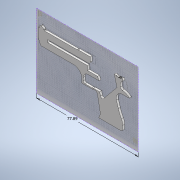
# Autodesk Inventor part: sheetmettaal_3
Saved by Autodesk Inventor 2022 (Build 260153000, 153)
## iProperties
Created: 2022-05-17
Part Number: sheetmettaal_3
Material: Generic
Document SubType Name: Sheet Metal
Designer: joshn
Density: 1 g/cm^3
Sheet Metal Rule: Default
Appearance: Default
Author: joshn
Autodesk Inventor part; units mm, degrees
ref_plane "YZ Plane" through (0, 0, 0) normal (1, 0, 0) x (0, 1, 0)
ref_plane "XZ Plane" through (0, 0, 0) normal (0, 1, 0) x (-1, 0, 0)
ref_plane "XY Plane" through (0, 0, 0) normal (0, 0, 1) x (1, 0, 0)
sketch "Sketch1" plane through (0, 0, 0) normal (0, 0, 1) x (1, 0, 0)
  line L0 (-5.5577, 9.6078) -> (72.3328, 9.6078) construction
  line L1 (72.3328, 9.6078) -> (72.3328, -46.9428) construction
  line L2 (72.3328, -46.9428) -> (-5.5577, -46.9428) construction
  line L3 (-5.5577, -46.9428) -> (-5.5577, 9.6078) construction
  point P0 (0, 0)
  dimension "d5" = 77.8905
  constraints: 1 vertical, 2 other
  measures "d5" distance of L1.end L2.end
sketch "Sketch2" plane through (0, 0, 0) normal (0, 0, 1) x (1, 0, 0)
  line L0 (1.7056, -0.1629) -> (1.7056, -0.6448)
  line L1 (-0.2664, 1.0493) -> (1.7056, -0.1629)
  line L2 (-0.7081, 1.0493) -> (-0.2664, 1.0493)
  arc A0 (-0.7081, 1.0493) -> (-1.4304, 0.327) centre (-0.7081, 0.327) ccw
  line L3 (-1.4304, -0.6448) -> (-1.4304, 0.327)
  line L4 (-2.6284, -0.6448) -> (-1.4304, -0.6448)
  line L5 (-2.6284, -7.7818) -> (-2.6284, -0.6448)
  line L6 (-0.8006, -12.1348) -> (-2.6284, -7.7818)
  line L7 (24.2675, -12.1348) -> (-0.8006, -12.1348)
  arc A1 (30.5055, -20.6992) -> (24.2675, -12.1348) centre (24.2675, -18.6888) ccw
  arc A2 (30.5055, -20.6992) -> (30.9333, -21.2865) centre (30.9333, -20.837) ccw
  line L8 (38.8712, -21.2865) -> (30.9333, -21.2865)
  line L9 (39.963, -20.923) -> (38.8712, -21.2865)
  arc A3 (42.6776, -22.7746) -> (39.963, -20.923) centre (40.3948, -23.2056) ccw
  line L10 (44.7723, -33.868) -> (42.6776, -22.7746)
  arc A4 (44.6306, -35.2789) -> (44.7723, -33.868) centre (42.2371, -34.3259) ccw
  line L11 (43.6296, -37.7931) -> (44.6306, -35.2789)
  line L12 (60.3255, -37.7931) -> (43.6296, -37.7931)
  line L13 (61.654, -37.1914) -> (60.3255, -37.7931)
  line L14 (61.8533, -33.7276) -> (61.654, -37.1914)
  arc A5 (61.8533, -33.7276) -> (60.9528, -29.7747) centre (54.5674, -33.3084) ccw
  arc A6 (58.6016, -24.1894) -> (60.9528, -29.7747) centre (85.7758, -16.0378) ccw
  line L15 (57.1367, -19.3061) -> (58.6016, -24.1894)
  arc A7 (61.717, -13.1502) -> (57.1367, -19.3061) centre (61.717, -17.9321) ccw
  line L16 (66.961, -13.1502) -> (61.717, -13.1502)
  arc A8 (66.961, -13.1502) -> (67.0884, -12.7993) centre (66.961, -12.9516) ccw
  arc A9 (67.0884, -12.7993) -> (61.7511, -10.5268) centre (60.666, -20.479) ccw
  arc A10 (60.1291, -9.1346) -> (61.7511, -10.5268) centre (61.9561, -8.647) ccw
  line L17 (59.0096, -4.9406) -> (60.1291, -9.1346)
  line L18 (55.449, -1.3577) -> (59.0096, -4.9406)
  line L19 (55.0519, -1.3577) -> (55.449, -1.3577)
  line L20 (57.6035, -10.735) -> (55.0519, -1.3577)
  line L21 (47.2749, -23.2615) -> (57.6035, -10.735)
  arc A11 (44.98, -22.7627) -> (47.2749, -23.2615) centre (46.2559, -22.4213) ccw
  line L22 (44.3049, -20.2402) -> (44.98, -22.7627)
  line L23 (33.0348, -20.5092) -> (36.1776, -20.5092)
  arc A12 (31.7579, -19.2323) -> (33.0348, -20.5092) centre (33.0348, -19.2323) ccw
  line L24 (31.7579, -17.0038) -> (31.7579, -19.2323)
  arc A13 (35.6115, -13.1502) -> (31.7579, -17.0038) centre (35.6115, -17.0038) ccw
  line L25 (36.1776, -13.1502) -> (35.6115, -13.1502)
  line L26 (42.6776, -10.735) -> (43.2318, -11.9426)
  line L27 (35.0069, -10.735) -> (42.6776, -10.735)
  line L28 (35.0069, -7.4885) -> (35.0069, -8.7654)
  line L29 (4.6149, -7.4885) -> (35.0069, -7.4885)
  line L30 (4.6149, -5.519) -> (4.6149, -7.4885)
  line L31 (35.7041, -5.519) -> (4.6149, -5.519)
  arc A14 (35.7041, -5.519) -> (37.089, -4.1341) centre (35.7041, -4.1341) ccw
  line L32 (37.089, -0.6448) -> (37.089, -4.1341)
  line L33 (28.0126, -0.6448) -> (37.089, -0.6448)
  arc A15 (27.0697, -0.9635) -> (28.0126, -0.6448) centre (27.0697, 0.5907) ccw
  line L34 (2.5258, -0.9635) -> (27.0697, -0.9635)
  arc A16 (1.9301, -0.6448) -> (2.5258, -0.9635) centre (2.5258, -0.2474) ccw
  line L35 (1.7056, -0.6448) -> (1.9301, -0.6448)
  arc A17 (38.0809, -13.3042) -> (39.1907, -13.9041) centre (40.5158, -10.1262) ccw
  arc A18 (38.0809, -13.3042) -> (37.6267, -13.1502) centre (37.6267, -13.897) ccw
  arc A19 (35.6115, -13.1502) -> (31.7579, -17.0038) centre (35.6115, -17.0038) ccw
  line L36 (31.7579, -17.0038) -> (31.7579, -19.2323)
  arc A20 (31.7579, -19.2323) -> (33.0348, -20.5092) centre (33.0348, -19.2323) ccw
  line L37 (33.0348, -20.5092) -> (38.3118, -20.5092)
  arc A21 (38.3118, -20.5092) -> (40.4901, -19.6055) centre (38.3087, -17.4247) ccw
  arc A22 (40.4901, -19.6055) -> (39.1907, -13.9041) centre (38.0474, -17.1634) ccw
  line L38 (37.089, -0.6448) -> (28.0126, -0.6448)
  line L39 (37.089, -4.1341) -> (37.089, -0.6448)
  arc A23 (35.7041, -5.519) -> (37.089, -4.1341) centre (35.7041, -4.1341) ccw
  line L40 (4.6149, -5.519) -> (35.7041, -5.519)
  line L41 (4.6149, -7.4885) -> (4.6149, -5.519)
  line L42 (35.0069, -7.4885) -> (4.6149, -7.4885)
  line L43 (35.0069, -8.7654) -> (35.0069, -7.4885)
  line L44 (57.6035, -10.735) -> (35.0069, -10.735)
  line L45 (55.0519, -1.3577) -> (57.6035, -10.735)
  line L46 (55.449, -1.3577) -> (55.0519, -1.3577)
  line L47 (59.0096, -4.9406) -> (55.449, -1.3577)
  line L48 (60.1291, -9.1346) -> (59.0096, -4.9406)
  arc A24 (60.1291, -9.1346) -> (61.7511, -10.5268) centre (61.9561, -8.647) ccw
  arc A25 (67.0884, -12.7993) -> (61.7511, -10.5268) centre (60.666, -20.479) ccw
  arc A26 (66.961, -13.1502) -> (67.0884, -12.7993) centre (66.961, -12.9516) ccw
  line L49 (61.717, -13.1502) -> (66.961, -13.1502)
  arc A27 (61.717, -13.1502) -> (57.1367, -19.3061) centre (61.717, -17.9321) ccw
  line L50 (58.6016, -24.1894) -> (57.1367, -19.3061)
  arc A28 (58.6016, -24.1894) -> (60.9528, -29.7747) centre (85.7758, -16.0378) ccw
  arc A29 (61.8533, -33.7276) -> (60.9528, -29.7747) centre (54.5674, -33.3084) ccw
  line L51 (61.654, -37.1914) -> (61.8533, -33.7276)
  line L52 (60.3255, -37.7931) -> (61.654, -37.1914)
  line L53 (43.6296, -37.7931) -> (60.3255, -37.7931)
  line L54 (44.6306, -35.2789) -> (43.6296, -37.7931)
  arc A30 (44.6306, -35.2789) -> (44.7723, -33.868) centre (42.2371, -34.3259) ccw
  line L55 (42.6776, -22.7746) -> (44.7723, -33.868)
  arc A31 (42.6776, -22.7746) -> (39.963, -20.923) centre (40.3948, -23.2056) ccw
  line L56 (38.8712, -21.2865) -> (39.963, -20.923)
  line L57 (30.9333, -21.2865) -> (38.8712, -21.2865)
  arc A32 (30.5055, -20.6992) -> (30.9333, -21.2865) centre (30.9333, -20.837) ccw
  arc A33 (30.5055, -20.6992) -> (24.2675, -12.1348) centre (24.2675, -18.6888) ccw
  line L58 (-0.8006, -12.1348) -> (24.2675, -12.1348)
  line L59 (-2.6284, -7.7818) -> (-0.8006, -12.1348)
  line L60 (-2.6284, -0.6448) -> (-2.6284, -7.7818)
  arc A34 (1.9301, -0.6448) -> (2.5258, -0.9635) centre (2.5258, -0.2474) ccw
  line L61 (27.0697, -0.9635) -> (2.5258, -0.9635)
  arc A35 (27.0697, -0.9635) -> (28.0126, -0.6448) centre (27.0697, 0.5907) ccw
  line L62 (44.3049, -20.2402) -> (40.49, -20.2402)
  line L63 (44.3049, -20.2402) -> (40.49, -20.2402)
  line L64 (40.49, -20.2402) -> (39.5685, -20.2402)
  line L65 (35.0069, -8.7654) -> (35.0069, -10.735)
  line L66 (35.6115, -13.1502) -> (43.786, -13.1502)
  line L67 (43.2318, -11.9426) -> (43.786, -13.1502)
  point P0 (0, 0)
extrude "Plate1" add sketch "Sketch2" along normal blind 1.5 contours L0 L35 A16 L34 A15 L33 L32 A14 L31 L30 L29 L28 L65 L27 L26 L67 L66 L25 A13 L24 A12 L23 L37 A21 L64 L62 L22 A11 L21 L20 L19 L18 L17 A10 A9 A8 L16 A7 L15 A6 A5 L14 L13 L12 L11 A4 L10 A3 L9 L8 A2 A1 L7 L6 L5 L4 L3 A0 L2 L1
sketch "Sketch3" plane through (0, 0, 0) normal (0, 0, -1) x (-1, 0, 0)
  line L0 (-60.1291, -9.1346) -> (-59.0096, -4.9406)
  line L1 (-59.0096, -4.9406) -> (-55.449, -1.3577)
  line L2 (-1.7056, -0.6448) -> (-1.7056, -0.1629)
  line L3 (-1.9301, -0.6448) -> (-1.7056, -0.6448)
  arc A0 (-2.5258, -0.9635) -> (-1.9301, -0.6448) centre (-2.5258, -0.2474) ccw
  line L4 (-27.0697, -0.9635) -> (-2.5258, -0.9635)
  arc A1 (-28.0126, -0.6448) -> (-27.0697, -0.9635) centre (-27.0697, 0.5907) ccw
  line L5 (-37.089, -0.6448) -> (-28.0126, -0.6448)
  line L6 (-37.089, -4.1341) -> (-37.089, -0.6448)
  arc A2 (-37.089, -4.1341) -> (-35.7041, -5.519) centre (-35.7041, -4.1341) ccw
  line L7 (-4.6149, -5.519) -> (-35.7041, -5.519)
  line L8 (-4.6149, -7.4885) -> (-4.6149, -5.519)
  line L9 (-35.0069, -7.4885) -> (-4.6149, -7.4885)
  line L10 (-35.0069, -8.7654) -> (-35.0069, -7.4885)
  line L11 (-4.6149, -8.7654) -> (-35.0069, -8.7654)
  line L12 (-4.6149, -10.735) -> (-4.6149, -8.7654)
  line L13 (-42.6776, -10.735) -> (-4.6149, -10.735)
  line L14 (-43.2318, -11.9426) -> (-42.6776, -10.735)
  line L15 (-36.1776, -11.9426) -> (-43.2318, -11.9426)
  line L16 (-36.1776, -13.1502) -> (-36.1776, -11.9426)
  line L17 (-35.6115, -13.1502) -> (-36.1776, -13.1502)
  arc A3 (-31.7579, -17.0038) -> (-35.6115, -13.1502) centre (-35.6115, -17.0038) ccw
  line L18 (-31.7579, -19.2323) -> (-31.7579, -17.0038)
  arc A4 (-33.0348, -20.5092) -> (-31.7579, -19.2323) centre (-33.0348, -19.2323) ccw
  line L19 (-36.1776, -20.5092) -> (-33.0348, -20.5092)
  line L20 (-36.1776, -20.8978) -> (-36.1776, -20.5092)
  line L21 (-38.5853, -20.8717) -> (-36.1776, -20.8978)
  arc A5 (-40.49, -20.2402) -> (-38.5853, -20.8717) centre (-38.5495, -17.5752) ccw
  line L22 (-44.3049, -20.2402) -> (-40.49, -20.2402)
  line L23 (-44.98, -22.7627) -> (-44.3049, -20.2402)
  arc A6 (-47.2749, -23.2615) -> (-44.98, -22.7627) centre (-46.2559, -22.4213) ccw
  line L24 (-57.6035, -10.735) -> (-47.2749, -23.2615)
  line L25 (-55.0519, -1.3577) -> (-57.6035, -10.735)
  line L26 (-55.449, -1.3577) -> (-55.0519, -1.3577)
  line L27 (-57.6171, -3.5394) -> (-55.449, -1.3577)
  arc A7 (-57.6171, -3.5394) -> (-58.5782, -3.3729) centre (-58.234, -4.243) ccw
  line L28 (-58.7548, -3.6332) -> (-58.5782, -3.3729)
  line L29 (-58.8916, -3.3186) -> (-58.7548, -3.6332)
  line L30 (-59.0682, -3.5789) -> (-58.8916, -3.3186)
  line L31 (-59.205, -3.2643) -> (-59.0682, -3.5789)
  line L32 (-59.3816, -3.5246) -> (-59.205, -3.2643)
  line L33 (-59.5184, -3.21) -> (-59.3816, -3.5246)
  line L34 (-59.695, -3.4703) -> (-59.5184, -3.21)
  line L35 (-59.8453, -3.1534) -> (-59.695, -3.4703)
  line L36 (-60.0219, -3.4136) -> (-59.8453, -3.1534)
  line L37 (-60.1298, -3.1041) -> (-60.0219, -3.4136)
  line L38 (-60.3064, -3.3644) -> (-60.1298, -3.1041)
  line L39 (-60.4432, -3.0498) -> (-60.3064, -3.3644)
  line L40 (-60.6198, -3.3101) -> (-60.4432, -3.0498)
  line L41 (-60.7566, -2.9955) -> (-60.6198, -3.3101)
  line L42 (-61.3674, -2.9657) -> (-60.7566, -2.9955)
  arc A8 (-61.3674, -2.9657) -> (-61.8521, -4.3697) centre (-61.4052, -3.7383) ccw
  arc A9 (-60.1291, -9.1346) -> (-61.8521, -4.3697) centre (-64.4153, -7.9905) ccw
  arc A10 (-61.7511, -10.5268) -> (-60.1291, -9.1346) centre (-61.9561, -8.647) ccw
  arc A11 (-61.7511, -10.5268) -> (-67.0884, -12.7993) centre (-60.666, -20.479) ccw
  arc A12 (-67.0884, -12.7993) -> (-66.961, -13.1502) centre (-66.961, -12.9516) ccw
  line L43 (-61.717, -13.1502) -> (-66.961, -13.1502)
  arc A13 (-57.1367, -19.3061) -> (-61.717, -13.1502) centre (-61.717, -17.9321) ccw
  line L44 (-58.6016, -24.1894) -> (-57.1367, -19.3061)
  arc A14 (-60.9528, -29.7747) -> (-58.6016, -24.1894) centre (-85.7758, -16.0378) ccw
  arc A15 (-60.9528, -29.7747) -> (-61.8533, -33.7276) centre (-54.5674, -33.3084) ccw
  line L45 (-61.654, -37.1914) -> (-61.8533, -33.7276)
  line L46 (-60.3255, -37.7931) -> (-61.654, -37.1914)
  line L47 (-43.6296, -37.7931) -> (-60.3255, -37.7931)
  line L48 (-44.6306, -35.2789) -> (-43.6296, -37.7931)
  arc A16 (-44.7723, -33.868) -> (-44.6306, -35.2789) centre (-42.2371, -34.3259) ccw
  line L49 (-42.6776, -22.7746) -> (-44.7723, -33.868)
  arc A17 (-39.963, -20.923) -> (-42.6776, -22.7746) centre (-40.3948, -23.2056) ccw
  line L50 (-38.8712, -21.2865) -> (-39.963, -20.923)
  line L51 (-30.9333, -21.2865) -> (-38.8712, -21.2865)
  arc A18 (-30.9333, -21.2865) -> (-30.5055, -20.6992) centre (-30.9333, -20.837) ccw
  arc A19 (-24.2675, -12.1348) -> (-30.5055, -20.6992) centre (-24.2675, -18.6888) ccw
  line L52 (0.8006, -12.1348) -> (-24.2675, -12.1348)
  line L53 (2.6284, -7.7818) -> (0.8006, -12.1348)
  line L54 (2.6284, -0.6448) -> (2.6284, -7.7818)
  line L55 (1.4304, -0.6448) -> (2.6284, -0.6448)
  line L56 (1.4304, 0.327) -> (1.4304, -0.6448)
  arc A20 (1.4304, 0.327) -> (0.7081, 1.0493) centre (0.7081, 0.327) ccw
  line L57 (0.2664, 1.0493) -> (0.7081, 1.0493)
  line L58 (-1.7056, -0.1629) -> (0.2664, 1.0493)
  point P0 (0, 0)
sheet face with bend "Face2" sketch "Sketch3" thickness 1.5 toward (0, 0, 1) bend radius 1.5 relief straight relief width 1.5 relief depth 0.75 contours A9 A8 L42 L41 L40 L39 L38 L37 L36 L35 L34 L33 L32 L31 L30 L29 L28 A7 L1 L0
bend "Bend1"
sketch "Sketch4" plane through (0, 0, 1.5) normal (0, 0, 1) x (1, 0, 0)
  line L0 (55.0519, -1.3577) -> (55.449, -1.3577) projected
  line L1 (55.4847, -2.9483) -> (55.0519, -1.3577) projected
  line L2 (57.0297, -2.9483) -> (55.4847, -2.9483) projected
  line L3 (55.449, -1.3577) -> (57.0297, -2.9483) projected
  point P0 (0, 0)
extrude "Cut1" cut sketch "Sketch4" against normal blind 1.5
equation "\"d23\" = Thickness"
equation "\"d16\" = Thickness"
equation "\"d18\" = BendRadius"
equation "\"d19\" = BendReliefWidth"
equation "\"d21\" = MinimumRemnant"
equation "\"d20\" = BendReliefDepth"
equation "\"d22\" = TransitionRadius"
equation "\"BendRadius\" = Thickness"
equation "\"BendReliefWidth\" = Thickness"
equation "\"BendReliefDepth\" = 0.5 * Thickness"
equation "\"CornerReliefSize\" = 4 * Thickness"
equation "\"MinimumRemnant\" = 2 * Thickness"
equation "\"TransitionRadius\" = BendRadius"
equation "\"JacobiRadiusSize\" = BendRadius"
equation "\"GapSize\" = Thickness"
equation "\"Thickness\" = 1.5"
body "Solid1"
